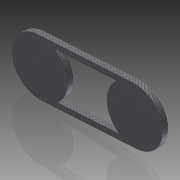
# Autodesk Inventor part: shooterchain
Saved by Autodesk Inventor 2011 SP1 (Build 150282100, 282)
## iProperties
Created: 2012-01-20
Part Number: shooterchain
Document SubType Name: Modeling
Designer: Christopher
Density: 1 g/cm^3
Author: Christopher
Autodesk Inventor part; units mm, degrees
ref_plane "YZ Plane" through (0, 0, 0) normal (1, 0, 0) x (0, 1, 0)
ref_plane "XZ Plane" through (0, 0, 0) normal (0, 1, 0) x (-1, 0, 0)
ref_plane "XY Plane" through (0, 0, 0) normal (0, 0, 1) x (1, 0, 0)
sketch "Sketch1" plane through (0, 0, 0) normal (0, 0, 1) x (1, 0, 0)
  circle A0 centre (17.9784, 0) radius 31.75
  circle A1 centre (125.9284, 6.35) radius 31.75
  line L0 (124.0639, 38.0452) -> (16.1139, 31.6952)
  line L1 (19.8428, -31.6952) -> (127.7928, -25.3452)
  line L2 (35.504, 26.4748) -> (105.4197, 30.5875)
  line L3 (108.4028, -20.1248) -> (38.487, -24.2375)
  line L4 (35.504, 26.4748) -> (16.1139, 31.6952)
  line L5 (38.487, -24.2375) -> (17.9784, -31.75)
  line L6 (108.4028, -20.1248) -> (127.7928, -25.3452)
  line L7 (105.4197, 30.5875) -> (124.0639, 38.0452)
  point P0 (0, 0)
  dimension "d0" = 107.95
  dimension "d1" = 6.35
  dimension "d2" = 63.5
  dimension "d3" = 63.5
  dimension "d4" = 6.35
  dimension "d5" = 6.35
  constraints: 16 end point, 11 point on circle, 3 parallel, 3 tangent, 2 centre point, 2 coincident, 2 point on line
  measures "d0" horizontal distance of point (125.928, 6.35) point (17.978, 0)
  measures "d1" vertical distance of point (17.978, 0) point (125.928, 6.35)
  measures "d2" diameter of A0
  measures "d3" diameter of A1
  measures "d4" distance between parallel lines of L1 L3
  measures "d5" distance between parallel lines of L0 L2
extrude "Extrusion1" add sketch "Sketch1" against normal blind 6.35 contours A0 L5 L4 | L4 A0 | A0 L0 A1 L2 | L3 A1 L1 A0 | A0 L5 | L7 A1 L6 | A1 L7 | L6 A1
body "Solid1"
